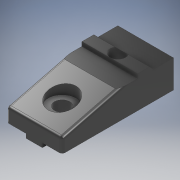
# Autodesk Inventor part: Y-Axis_Extursion_Mount_LM3041
Saved by Autodesk Inventor 2020.3 (Build 243373000, 373)
## iProperties
Created: 2020-05-30
Part Number: Y-Axis_Extursion_Mount_LM3041
Material: ABS Plastic
Document SubType Name: Modeling
Designer: rah75
Density: 1.06 g/cm^3
Appearance: Satin - Black
Author: rah75
Autodesk Inventor part; units mm, degrees
ref_plane "YZ Plane" through (0, 0, 0) normal (1, 0, 0) x (0, 1, 0)
ref_plane "XZ Plane" through (0, 0, 0) normal (0, 1, 0) x (-1, 0, 0)
ref_plane "XY Plane" through (0, 0, 0) normal (0, 0, 1) x (1, 0, 0)
sketch "Sketch1" plane through (0, 0, 0) normal (1, 0, 0) x (0, 1, 0)
  line L0 (0, 0) -> (10, 0)
  line L1 (10, 0) -> (10, 20)
  line L2 (10, 20) -> (5, 40)
  line L3 (5, 40) -> (0, 40)
  line L4 (0, 40) -> (0, 0)
  dimension "d0" = 10
  dimension "d1" = 5
  dimension "d2" = 20
  dimension "d3" = 20
  constraints: 10 end point, 2 perpendicular, 1 horizontal, 1 parallel
  measures "d0" distance of L0.start L0.end
  measures "d1" distance of L2.end L3.end
  measures "d2" distance of L0.end L1.end
  measures "d3" distance from line of L1.end L3
extrude "Extrusion1" add sketch "Sketch1" along normal mid plane 20
sketch "Sketch2" plane through (-10, 0, 40) normal (0, 0, 1) x (1, 0, 0)
  line L0 (7.1, -1.5) -> (12.9, -1.5)
  line L1 (12.9, -1.5) -> (12.9, 0)
  line L2 (12.9, 0) -> (7.1, 0)
  line L3 (7.1, 0) -> (7.1, -1.5)
  line L4 (7.1, -1.5) -> (12.9, 0) construction
  line L5 (12.9, -1.5) -> (7.1, 0) construction
  line L6 (0, 0) -> (20, 0) projected
  point P0 (10, 0)
  point P1 (10, -0.75)
  point P2 (10, 0)
  dimension "d6" = 5.8
  dimension "d7" = 1.5
  constraints: 12 end point, 4 midpoint, 2 parallel, 1 horizontal, 1 perpendicular
  measures "d6" distance of L0.start L0.end
  measures "d7" distance of L0.end L1.end
extrude "Extrusion2" add sketch "Sketch2" against normal up to surface (40 mm away)
sketch "Sketch5" plane through (10, 0, 0) normal (1, 0, 0) x (0, 0, -1)
  line L0 (-12.875, 11.5) -> (-7.125, 11.5)
  line L1 (-7.125, 11.5) -> (-7.125, 10)
  line L2 (-7.125, 10) -> (-12.875, 10)
  line L3 (-12.875, 10) -> (-12.875, 11.5)
  line L4 (-12.875, 11.5) -> (-7.125, 10) construction
  line L5 (-7.125, 11.5) -> (-12.875, 10) construction
  line L6 (0, 10) -> (-20, 10) projected
  point P0 (0, 0)
  point P1 (-10, 10.75)
  point P2 (-10, 10)
  dimension "d24" = 5.75
  dimension "d25" = 1.5
  constraints: 12 end point, 4 midpoint, 2 parallel, 1 horizontal, 1 perpendicular
  measures "d24" distance of L1.end L2.end
  measures "d25" distance of L0.end L1.end
extrude "Extrusion3" add sketch "Sketch5" against normal up to surface (20 mm away)
chamfer "Chamfer1" distance 1.5 angle 45 1 edges at (0, 11.5, 7.125)
sketch "Sketch3" plane through (-10, 10, 20) normal (0, 1, 0) x (1, 0, 0)
  line L0 (0, -20) -> (20, -20) projected
  line L1 (20, 0) -> (20, -20) projected
  line L2 (0, 0) -> (20, 0) projected
  line L3 (0, -20) -> (0, 0) projected
  point P0 (10, 20)
  point P1 (10, -10)
  point P2 (10, 0)
  point P3 (0, -10)
  constraints: 2 midpoint, 1 horizontal alignment, 1 vertical alignment
hole "Hole1" at (0, 10, 30) direction (0, -1, 0) diameter 5.5 end through all start extended yes counterbore diameter 10 counterbore depth 5 clearance for "Socket Head Cap Screw" size "M5" standard "Ansi Metric M Profile"
sketch "Sketch4" plane through (-2.9, -1.5, 40) normal (0, -1, 0) x (1, 0, 0)
  line L0 (-7.1, -20) -> (12.9, -20) projected
  line L1 (12.9, -40) -> (12.9, -32.875) projected
  line L2 (12.9, -40) -> (-7.1, -40) projected
  line L3 (-7.1, -20) -> (-7.1, -27.125) projected
  line L4 (-7.1, -32.875) -> (12.9, -32.875) projected
  line L5 (-7.1, -32.875) -> (-7.1, -40) projected
  line L6 (12.9, -27.125) -> (-7.1, -27.125) projected
  line L7 (12.9, -27.125) -> (12.9, -20) projected
  point P0 (2.9, -40)
  point P1 (2.9, -30)
  point P2 (-7.1, -30)
  point P3 (2.9, -20)
  constraints: 1 horizontal alignment, 1 midpoint, 1 point on line, 1 vertical alignment
hole "Hole2" at (0, -1.5, 10) direction (0, 1, 0) diameter 5.5 end through all start extended yes counterbore diameter 10 counterbore depth 7.25 clearance for "Socket Head Cap Screw" size "M5" standard "Ansi Metric M Profile"
fillet "Fillet1" radius 1 5 edges at (0, 5, 40) (-10, 7.5, 30) (10, 7.5, 30) (10, 2.5, 40) (-10, 2.5, 40)
body "Solid1"
